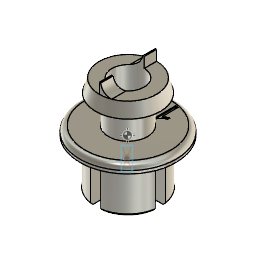
закрутка12 шлиц v9 v1 (Autodesk Fusion 360 design; units mm, degrees)
Autodesk Fusion 360 part; units mm, degrees
sketch "Sketch1" plane through (0, 0, 0) normal (0, 1, 0) x (1, 0, 0)
  line L0 (6.2, -37.4) -> (11, -37.4)
  line L1 (11, -37.4) -> (12.4, -32.4)
  line L2 (12.4, -32.4) -> (7.5, -31)
  line L3 (7.5, -31) -> (7.5, -21.6)
  line L4 (7.5, -21.6) -> (16.5, -21.6)
  line L5 (18.5, -19.6) -> (18.5, -18.5)
  line L6 (18.5, -18.5) -> (13.75, -18.5)
  line L7 (13.75, -18.5) -> (13.75, -18)
  line L8 (13.75, -18) -> (12.59, -18)
  line L9 (12.59, -18) -> (12.59, -15)
  line L10 (12.59, -15) -> (12.6, -15)
  line L11 (12.6, -15) -> (12.6, -1)
  line L12 (11.6, 0) -> (8.2, 0)
  line L13 (6.2, -37.4) -> (6.2, -14)
  line L14 (7.2, -1) -> (7.2, -13)
  line L15 (8.2, 0) -> (7.2, -1)
  line L16 (7.2, -13) -> (6.2, -14)
  arc A0 (16.5, -21.6) -> (18.5, -19.6) centre (16.5, -19.6) ccw
  line L17 (11.6, 0) -> (12.6, -1)
  point P0 (18.5, -21.6)
  dimension "d3" = 12.4
  dimension "d9" = 3
  dimension "d10" = 0.5
  dimension "d11" = 3.1
  dimension "d12" = 10.8
  dimension "d13" = 9.4
  dimension "d16" = 6.2
  dimension "d17" = 8.2
  dimension "d18" = 7.2
  dimension "d19" = 1
  dimension "d20" = 1
  dimension "d21" = 13
  dimension "d22" = 11
  dimension "d24" = 13.75
  dimension "d25" = 18.5
  dimension "d26" = 7.5
  dimension "d27" = 12.59
  dimension "d28" = 2
  dimension "d29" = 37.4
  dimension "d79" = 1
  dimension "d81" = 1
  dimension "d82" = 15
  dimension "d83" = 12.6
  constraint perpendicular L0 L3
  constraint perpendicular L3 L4
  constraint perpendicular L0 L5
  constraint perpendicular L5 L6
  constraint perpendicular L6 L7
  constraint perpendicular L7 L8
  constraint perpendicular L8 L9
  constraint perpendicular L7 L10
  constraint perpendicular L10 L11
  constraint horizontal L12
  constraint perpendicular L12 L13
  constraint perpendicular L12 L14
  constraint coincident P0 L4
  constraint coincident P0 L5
  constraint tangent L4 A0
  constraint tangent L5 A0
  constraint vertical L3
  measures "d3" horizontal distance of origin L1.end
  measures "d9" distance of L8.end L9.end
  measures "d10" distance of L6.end L7.end
  measures "d11" distance of P0 L5.end
  measures "d12" distance of L1.end L4
  measures "d13" distance of L2.end L4
  measures "d16" distance of origin L13
  measures "d17" distance of origin L12.end
  measures "d18" horizontal distance of origin L14.start
  measures "d19" vertical distance of L14.end L13.end
  measures "d20" vertical distance of L12.end L14.start
  measures "d21" vertical distance of origin L14.end
  measures "d22" horizontal distance of origin L0.end
  measures "d24" horizontal distance of origin L7.end
  measures "d25" horizontal distance of origin P0
  measures "d26" distance of origin L3
  measures "d27" horizontal distance of origin L9.end
  measures "d28" radius of A0
  measures "d29" vertical distance of origin L0.start
  measures "d79" horizontal distance of L12.start L11.end
  measures "d81" vertical distance of L12.start L11.end
  measures "d82" vertical distance of origin L10.end
  measures "d83" horizontal distance of origin L11.end
revolve "Revolve2" add sketch "Sketch1" angle 360 about axis through (0, 0, 1.75) along (0, 0, 1) makes body 1
sketch "Sketch2" plane through (0, 0, 0) normal (0, 0, -1) x (1, 0, 0)
  circle A0 centre (0, 0) radius 8.2
  circle A1 centre (0, 0) radius 12.6
  line L0 (14, -2) -> (-14, -2)
  line L1 (-14, -2) -> (-14, 2)
  line L2 (-14, 2) -> (14, 2)
  line L3 (14, 2) -> (14, -2)
  line L4 (14, -2) -> (-14, 2) construction
  line L5 (-14, -2) -> (14, 2) construction
  line L6 (2, -15) -> (-2, -15)
  line L7 (-2, -15) -> (-2, 15)
  line L8 (-2, 15) -> (2, 15)
  line L9 (2, 15) -> (2, -15)
  line L10 (2, -15) -> (-2, 15) construction
  line L11 (-2, -15) -> (2, 15) construction
  dimension "d31" = 4
  dimension "d32" = 4
  constraint horizontal L0
  constraint perpendicular L0 L1
  constraint parallel L0 L2
  constraint parallel L1 L3
  constraint coincident L4 A0.centre
  constraint coincident L5 A0.centre
  constraint coincident A0.centre A1.centre
  constraint horizontal L6
  constraint perpendicular L6 L7
  constraint parallel L6 L8
  constraint parallel L7 L9
  constraint coincident L10 A0.centre
  constraint coincident L11 A0.centre
  measures "d31" distance of L7.end L8.end
  measures "d32" distance of L0.start L2.end
extrude "Extrude3" cut sketch "Sketch2" against normal blind 17 contours A0 L0 L2 L9 | A0 A1 L0 L2 | A0 L2 L7 L9 | A0 A1 L7 L9 | A0 A1 L7 L9 | A0 L0 L7 L9 | A0 L0 L2 L7 | A0 A1 L0 L2 bodies 1
fillet "Fillet1" radius 2 2 edges at (9.1493, 2, 17) (9.1493, -2, 17) on bodies 1
fillet "Fillet1" radius 2 6 edges at (2, -9.1493, 17) (-2, -9.1493, 17) (-2, 9.1493, 17) (2, 9.1493, 17) (-9.1493, 2, 17) (-9.1493, -2, 17) on bodies 1
sketch "Sketch4" plane through (0, 0, 37.4) normal (0, 0, 1) x (-1, 0, 0)
  circle A0 centre (0, 0) radius 11
  circle A1 centre (0, 0) radius 6.2
  circle A2 centre (0, 0) radius 6.2 construction
  circle A3 centre (0, 0) radius 11 construction
  line L0 (0, -13) -> (4, -13)
  line L1 (4, -13) -> (4, -2)
  line L2 (4, -2) -> (0, -2)
  line L3 (0, -2) -> (0, -13)
  constraint horizontal L0
  constraint vertical L1
  constraint horizontal L2
  constraint vertical L3
extrude "Extrude4" add sketch "Sketch4" along normal blind 4 contours A0 A1 L1 L3 picked at (2.8059, -8.9559) bodies 1
ref_plane "WorkPlane1" through (0, 11, 41.4) normal (0, 1, 0) x (-1, 0, 0)
sketch "Sketch5" plane through (0, 11, 0) normal (0, 1, 0) x (1, 0, 0)
  line L0 (-4, -41.4) -> (0, -41.4)
  line L1 (-4, -37.4) -> (-4, -41.4)
  arc A0 (-0.5, -41.4) -> (-4, -37.4) centre (-5.3686, -42.1288) ccw
  point P0 (-4, -41.4)
  constraint coincident L1.start A0.end
  constraint coincident L0 A0.start
extrude "Extrude5" cut sketch "Sketch5" against normal blind 7.5 bodies 1
pattern_circular "C-Pattern1" count 2 over 360 about axis through (0, 0, 1.75) along (0, 0, 1) of 4 faces at (-0.8641, 10.966, 38.0887) (-0.5921, 7.7751, 40.9375) (0, 7.8, 38.7333) (-0.1112, 7.7988, 41.4) on bodies 1
ref_plane "WorkPlane2" through (-9.1544, -2, 8.5) normal (0, 1, 0) x (-1, 0, 0)
sketch "Sketch6" plane through (0, -2, 0) normal (0, 1, 0) x (1, 0, 0)
  line L0 (-12.5, -11.2) -> (-12.8, -11.2)
  line L1 (-12.8, -11.2) -> (-12.8, -9.2)
  line L2 (-12.8, -9.2) -> (-12.5, -9.2)
  line L3 (-12.5, -9.2) -> (-12.5, -11.2)
  point P0 (-12.4403, 0)
  dimension "d56" = 9.2
  dimension "d57" = 2
  dimension "d58" = 0.3
  constraint horizontal L0
  constraint vertical L1
  constraint horizontal L2
  constraint vertical L3
  measures "d56" vertical distance of L2.end P0
  measures "d57" distance of L0.end L1.end
  measures "d58" distance of L0.start L0.end
revolve "Revolve3" add sketch "Sketch6" angle 70 about axis through (0, 0, 1.75) along (0, 0, 1) separate body makes body 2
pattern_circular "C-Pattern2" count 2 over 360 about axis through (0, 0, 1.75) along (0, 0, 1) of bodies 2 makes body 3
ref_plane "WorkPlane5" through (-2, 12.4403, 15) normal (0.707107, -0.707107, 0) x (0.707107, 0.707107, 0)
ref_plane "WorkPlane7" through (-5.3146, 4.8575, 6.0719) normal (0.738138, -0.67465, 0) x (-0.67465, -0.738138, 0)
sketch "Sketch9" plane through (-5.3146, 4.8575, 0) normal (0.738138, -0.67465, 0) x (-0.67465, -0.738138, 0)
  line L0 (1.5, -9.8489) -> (-1.5, -9.8489)
  line L1 (-1.5, -9.8489) -> (-1.5, -1.1511)
  line L2 (-1.5, -1.1511) -> (1.5, -1.1511)
  line L3 (1.5, -1.1511) -> (1.5, -9.8489)
  line L4 (1.5, -9.8489) -> (-1.5, -1.1511) construction
  line L5 (-1.5, -9.8489) -> (1.5, -1.1511) construction
  point P0 (0, -5.5)
  dimension "d85" = 3
  constraint horizontal L0
  constraint perpendicular L0 L1
  constraint parallel L0 L2
  constraint parallel L1 L3
  constraint coincident L4 P0
  constraint coincident L5 P0
  measures "d85" distance of L1.end L2.end
extrude "Extrude6" add sketch "Sketch9" along normal blind 2.2 separate body makes body 4
chamfer "Chamfer1" distance 1.4 angle 45 4 edges at (-2.6787, 4.4805, 5.5) (-4.7027, 2.266, 5.5) (-3.6907, 3.3732, 1.1511) (-3.6907, 3.3732, 9.8489) on bodies 4
pattern_circular "C-Pattern3" count 2 over 360 about axis through (0, 0, 1.75) along (0, 0, 1) of bodies 4 makes body 5
ref_plane "WorkPlane8" through (0, 0, 21.6) normal (0, 0, 1) x (1, 0, 0)
sketch "Sketch11" plane through (0, 0, 21.6) normal (0, 0, 1) x (1, 0, 0)
  line L0 (5.5832, 15.4015) -> (-5.8341, 15.2898) construction
  line L1 (-5.8341, 15.2898) -> (-5.7584, 7.5573) construction
  line L2 (-5.7584, 7.5573) -> (5.6588, 7.669) construction
  line L3 (5.6588, 7.669) -> (5.5832, 15.4015) construction
  dimension "d92" = 8
  text T0 "12" font "Arial" height 8 align left top in box 11.4178 x 7.7328 at (5.5832, 15.4015) x (-0.999952, -0.009782) y (0.009782, -0.999952) spacing 1 kerned
extrude "Extrude7" cut sketch "Sketch11" against normal blind 0.4 text T0 bodies 1
delete_body "RemoveBody1" bodies 2
delete_body "RemoveBody2" bodies 3
equation "d93 = 0 mm - 0.4 mm"
named bodies: "Шліц", "Шліц (1)"
